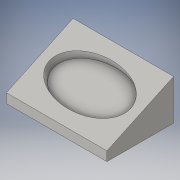
# Autodesk Inventor part: MonitorBase
Saved by Autodesk Inventor 2016 (Build 200138000, 138)
## iProperties
Created: 2015-08-27
Part Number: MonitorBase
Material: Generic
Document SubType Name: Modeling
Designer: steele
Density: 1 g/cm^3
Appearance: Default
Author: steele
Autodesk Inventor part; units mm, degrees
ref_plane "YZ Plane" through (0, 0, 0) normal (1, 0, 0) x (0, 1, 0)
ref_plane "XZ Plane" through (0, 0, 0) normal (0, 1, 0) x (-1, 0, 0)
ref_plane "XY Plane" through (0, 0, 0) normal (0, 0, 1) x (1, 0, 0)
sketch "Sketch1" plane through (0, 0, 0) normal (1, 0, 0) x (0, 1, 0)
  line L0 (0, -90.4875) -> (25.4, -90.4875)
  line L1 (25.4, -90.4875) -> (109.79, 90.4875)
  line L2 (109.79, 90.4875) -> (0, 90.4875)
  line L3 (0, 0) -> (0, 90.4875)
  line L4 (0, 0) -> (0, -90.4875)
  line L5 (109.79, 90.4875) -> (109.79, -90.4875) construction
  dimension "baseDepth" = 180.975
  dimension "tilt" = -25
  dimension "frontHeight" = 25.4
  constraints: 12 end point, 2 collinear, 1 parallel, 1 perpendicular, 1 point on line, 1 vertical
  measures "baseDepth" distance of L0.start L2.end
  measures "tilt" angle of L1 L5
  measures "frontHeight" distance of L0.start L0.end
extrude "Extrusion1" add sketch "Sketch1" along normal mid plane 273.05
sketch "Sketch5" plane through (-136.525, 109.79, 90.4875) normal (0, 0.9063, -0.4226) x (1, 0, 0)
  line L0 (273.05, 199.6838) -> (0, 199.6838) construction
  line L1 (273.05, 199.6838) -> (273.05, 0) construction
  line L2 (0, 199.6838) -> (273.05, 0) construction
  line L3 (273.05, 0) -> (0, 0) construction
  line L4 (273.05, 199.6838) -> (0, 0) construction
  ellipse E0 centre (136.525, 99.8419) end of major axis (247.65, 99.8419) minor radius 65.0875
  point P0 (136.525, 128.4088)
  dimension "elipseMajorRadius" = 111.125
  dimension "elipseMinorRadius" = 65.0875
  constraints: 4 end point, 1 midpoint, 2 other
extrude "Extrusion3" cut sketch "Sketch5" against normal blind 25.4
equation "\"tilt\" = -tiltAngle"
equation "\"elipseMajorRadius\" = 0.5 * monitorBaseElipseMajorDiam"
equation "\"elipseMinorRadius\" = 0.5 * monitorBaseElipseMinorDiam"
equation "\"monitorBaseElipseMajorDiam\" = 222.25"
equation "\"monitorBaseElipseMinorDiam\" = 130.175"
equation "\"tiltAngle\" = 25deg"
body "Solid1"
